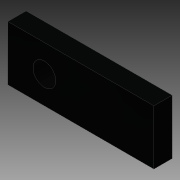
# Autodesk Inventor part: Weight_Bottom_Fixture
Saved by Autodesk Inventor 2015 (Build 190159000, 159)
## iProperties
Created: 2015-01-09
Part Number: Weight_Bottom_Fixture
Material: Aluminum, Anodized Black
Document SubType Name: Modeling
Designer: Drew
Density: 2.7 g/cm^3
Appearance: Anodized - Blue(1)
Author: Drew
Autodesk Inventor part; units mm, degrees
ref_plane "YZ Plane" through (0, 0, 0) normal (1, 0, 0) x (0, 1, 0)
ref_plane "XZ Plane" through (0, 0, 0) normal (0, 1, 0) x (-1, 0, 0)
ref_plane "XY Plane" through (0, 0, 0) normal (0, 0, 1) x (1, 0, 0)
sketch "Sketch1" plane through (0, 0, 0) normal (0, 0, 1) x (1, 0, 0)
  line L0 (50.8, -19.05) -> (-50.8, -19.05)
  line L1 (-50.8, -19.05) -> (-50.8, 19.05)
  line L2 (-50.8, 19.05) -> (50.8, 19.05)
  line L3 (50.8, 19.05) -> (50.8, -19.05)
  line L4 (50.8, -19.05) -> (-50.8, 19.05) construction
  line L5 (-50.8, -19.05) -> (50.8, 19.05) construction
  circle A0 centre (-25.4, 0) radius 7.9375
  point P0 (0, 0)
  dimension "d0" = 38.1
  dimension "d1" = 101.6
  dimension "d2" = 15.875
  dimension "d3" = 25.4
  constraints: 12 end point, 2 midpoint, 2 parallel, 1 centre point, 1 horizontal, 1 perpendicular
  measures "d0" distance of L0.end L1.end
  measures "d1" distance of L1.end L2.end
  measures "d2" diameter of A0
  measures "d3" distance from line of L1 A0.centre
extrude "Extrusion1" add sketch "Sketch1" along normal blind 12.7
equation "\"d0\" = Fixture_Width"
equation "\"d1\" = Fixture_Length"
equation "\"d2\" = Main_Shaft_Diameter"
equation "\"d4\" = Fixture_Thickness"
equation "\"Fixture_Width\" = 38.1"
equation "\"Fixture_Length\" = 101.6"
equation "\"Main_Shaft_Diameter\" = 15.875"
equation "\"Fixture_Thickness\" = 12.7"
body "Solid1"
